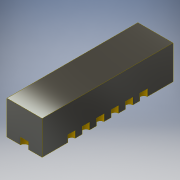
# Autodesk Inventor part: MC_HQ1157
Saved by Autodesk Inventor 2016 (Build 200138000, 138)
## iProperties
Created: 2016-08-30
Part Number: MC_HQ1157
Material: Generic
Document SubType Name: Modeling
Designer: jfixelle
Density: 1 g/cm^3
Appearance: Silver
Author: jfixelle
Autodesk Inventor part; units mm, degrees
ref_plane "YZ Plane" through (0, 0, 0) normal (1, 0, 0) x (0, 1, 0)
ref_plane "XZ Plane" through (0, 0, 0) normal (0, 1, 0) x (-1, 0, 0)
ref_plane "XY Plane" through (0, 0, 0) normal (0, 0, 1) x (1, 0, 0)
sketch "Sketch1" plane through (0, 0, 0) normal (0, 1, 0) x (-1, 0, 0)
  line L0 (4.635, 17.27) -> (-4.635, 17.27)
  line L1 (-4.635, 17.27) -> (-4.635, -17.27)
  line L2 (-4.635, -17.27) -> (4.635, -17.27)
  line L3 (4.635, -17.27) -> (4.635, 17.27)
  point P0 (0, 0)
  dimension "d0" = 9.27
  dimension "d1" = 4.635
  dimension "d2" = 34.54
  dimension "d3" = 17.27
  constraints: 8 end point, 2 parallel, 1 horizontal, 1 perpendicular
  measures "d0" distance of L1.end L2.end
  measures "d1" distance from line of point (0, 0) L3
  measures "d2" distance of L2.end L0.start
  measures "d3" distance from line of L2 point (0, 0)
extrude "Extrusion1" add sketch "Sketch1" along normal blind 8.89
sketch "Sketch2" plane through (0, 0, 0) normal (0, -1, 0) x (1, 0, 0)
  line L0 (4.685, 10.79) -> (2.145, 10.79)
  line L1 (2.145, 10.79) -> (2.145, 8.25)
  line L2 (2.145, 8.25) -> (4.685, 8.25)
  line L3 (4.685, 8.25) -> (4.685, 10.79)
  line L4 (4.635, 17.27) -> (4.635, -17.27) projected
  line L5 (-4.635, 17.27) -> (4.635, 17.27) projected
  circle A0 centre (4.685, 9.52) radius 0.9772
  point P0 (0, 0)
  dimension "d6" = 2.54
  dimension "d7" = 2.54
  dimension "d8" = 0.05
  dimension "d9" = 6.48
  constraints: 8 end point, 2 parallel, 1 centre point, 1 horizontal, 1 midpoint, 1 perpendicular
  measures "d6" distance of L2.end L0.start
  measures "d7" distance of L1.end L2.end
  measures "d8" distance between parallel lines of L4 L3
  measures "d9" distance between parallel lines of L5 L0
extrude "Extrusion2" cut sketch "Sketch2" against normal blind 1.778 contours A0 L3 | L3 A0 L4 | L4 A0
pattern_linear "Rectangular Pattern1" count 6 spacing 3.81 along (0, 0, -1) of "Extrusion2"
mirror "Mirror1" about plane through (0, 0, 0) normal (1, 0, 0) of "Extrusion2", "Rectangular Pattern1"
sketch "Sketch3" plane through (0, 0, 0) normal (0, -1, 0) x (1, 0, 0)
  line L0 (1.27, -14.78) -> (-1.27, -14.78)
  line L1 (-1.27, -14.78) -> (-1.27, -17.32)
  line L2 (-1.27, -17.32) -> (1.27, -17.32)
  line L3 (1.27, -17.32) -> (1.27, -14.78)
  line L4 (4.635, -17.27) -> (-4.635, -17.27) projected
  circle A0 centre (0, -17.32) radius 1.0823
  point P0 (0, 0)
  dimension "d15" = 2.54
  dimension "d16" = 1.27
  dimension "d17" = 2.54
  dimension "d18" = 0.05
  constraints: 8 end point, 2 parallel, 1 centre point, 1 horizontal, 1 midpoint, 1 perpendicular
  measures "d15" distance of L1.end L2.end
  measures "d16" distance from line of point (0, 0) L3
  measures "d17" distance of L2.end L0.start
  measures "d18" distance between parallel lines of L4 L2
extrude "Extrusion3" cut sketch "Sketch3" against normal blind 1.778 contours A0 L2 L4 | L4 A0 | A0 L2
mirror "Mirror2" about plane through (0, 0, 0) normal (0, 0, 1) of "Extrusion3"
body "Solid1"
